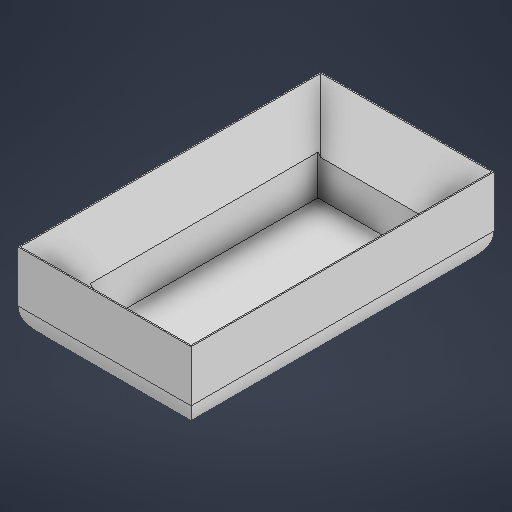
# Autodesk Inventor part: мыльница
Saved by Autodesk Inventor 2025 (Build 290162000, 162)
## iProperties
Created: 2024-12-03
Part Number: мыльница
Material: Типовые
Document SubType Name: Modeling
Designer: GameHD
Density: 1 g/cm^3
Appearance: По умолчанию
Author: GameHD
Autodesk Inventor part; units mm, degrees
ref_plane "YZ Plane" through (0, 0, 0) normal (1, 0, 0) x (0, 1, 0)
ref_plane "XZ Plane" through (0, 0, 0) normal (0, 1, 0) x (-1, 0, 0)
ref_plane "XY Plane" through (0, 0, 0) normal (0, 0, 1) x (1, 0, 0)
sketch "Эскиз1" plane through (0, 0, 0) normal (0, 0, 1) x (1, 0, 0)
  line L0 (-19.75, -19.75) -> (19.75, -19.75)
  line L1 (19.75, -19.75) -> (19.75, 19.75)
  line L2 (19.75, 19.75) -> (-19.75, 19.75)
  line L3 (-19.75, 19.75) -> (-19.75, -19.75)
  line L4 (-19.75, -19.75) -> (19.75, 19.75) construction
  line L5 (19.75, -19.75) -> (-19.75, 19.75) construction
  line L6 (-35, -35) -> (35, -35)
  line L7 (35, -35) -> (35, 35)
  line L8 (35, 35) -> (-35, 35)
  line L9 (-35, 35) -> (-35, -35)
  line L10 (-35, -35) -> (35, 35) construction
  line L11 (35, -35) -> (-35, 35) construction
  line L12 (-19.75, 19.75) -> (-35, 19.75)
  line L13 (19.75, 19.75) -> (35, 19.75)
  point P0 (0, 0)
  dimension "d0" = 39.5
  dimension "d1" = 39.5
  dimension "d2" = 70
  dimension "d3" = 70
  constraints: 28 end point, 4 midpoint, 4 parallel, 3 perpendicular, 3 point on line, 2 horizontal
  measures "d0" distance of L2.end L1.end
  measures "d1" distance of L1.end L0.end
  measures "d2" distance of L8.end L7.end
  measures "d3" distance of L8.end L6.start
extrude "Выдавливание1" add sketch "Эскиз1" along normal blind 92 contours L0 L1 L13 L7 L6 L9 L12 L3
sketch "Эскиз2" plane through (0, 0, 0) normal (0, 0, -1) x (-1, 0, 0)
  line L0 (-19.75, -19.75) -> (19.75, -19.75) projected
  line L1 (-19.75, 19.75) -> (-19.75, -19.75) projected
  line L2 (-35, 19.75) -> (-19.75, 19.75) projected
  line L3 (-35, -35) -> (-35, 19.75) projected
  line L4 (35, -35) -> (-35, -35) projected
  line L5 (35, 19.75) -> (35, -35) projected
  line L6 (19.75, 19.75) -> (35, 19.75) projected
  line L7 (19.75, -19.75) -> (19.75, 19.75) projected
  line L8 (-19.75, 19.75) -> (19.75, 19.75)
  point P0 (0, 0)
  constraints: 2 end point, 1 horizontal
extrude "Выдавливание2" add sketch "Эскиз2" along normal blind 15.25
sketch "Эскиз3" plane through (0, 0, 92) normal (0, 0, 1) x (1, 0, 0)
  line L0 (19.75, -19.75) -> (-19.75, -19.75) projected
  line L1 (-19.75, -19.75) -> (-19.75, 19.75) projected
  line L2 (-19.75, 19.75) -> (-35, 19.75) projected
  line L3 (-35, 19.75) -> (-35, -35) projected
  line L4 (-35, -35) -> (35, -35) projected
  line L5 (35, -35) -> (35, 19.75) projected
  line L6 (35, 19.75) -> (19.75, 19.75) projected
  line L7 (19.75, 19.75) -> (19.75, -19.75) projected
  line L8 (-19.75, 19.75) -> (19.75, 19.75) projected
  point P0 (0, 0)
extrude "Выдавливание3" add sketch "Эскиз3" along normal blind 15.25
sketch "Эскиз4" plane through (-35, -35, -15.25) normal (-1, 0, 0) x (0, 0, 1)
  line L0 (0, 54.75) -> (200, 54.75)
  line L1 (200, 54.75) -> (200, 44.75)
  line L2 (200, 44.75) -> (0, 44.75)
  line L3 (0, 44.75) -> (0, 54.75)
  dimension "d12" = 200
  dimension "d13" = 10
  constraints: 8 end point, 2 parallel, 1 horizontal, 1 perpendicular
  measures "d12" distance of L1.end L2.end
  measures "d13" distance of L0.end L1.end
extrude "Выдавливание4" cut sketch "Эскиз4" against normal through all
chamfer "Фаска1" distance 14.7625 angle 45 4 edges at (0, 9.75, 92) (19.75, 9.75, 46) (-19.75, 9.75, 46) (0, 9.75, 0)
sketch "Эскиз5" plane through (-35, -35, -15.25) normal (0, -1, 0) x (1, 0, 0)
  line L0 (70, 0) -> (70, 122.5) projected
  line L1 (0, 122.5) -> (70, 122.5) projected
  line L2 (0, 0) -> (0, 122.5) projected
  line L3 (70, 0) -> (0, 0) projected
  point P0 (35, 15.25)
extrude "Выдавливание5" cut sketch "Эскиз5" against normal blind 12.05
fillet "Сопряжение1" radius 12 4 edges at (35, -22.95, 46) (0, -22.95, 107.25) (0, -22.95, -15.25) (-35, -22.95, 46)
sketch "Эскиз6" plane through (-19.75, -19.75, 0) normal (0, 1, 0) x (1, 0, 0)
  line L0 (39.5, 0) -> (0, 0) projected
  line L1 (0, 0) -> (0, -92) projected
  line L2 (39.5, -92) -> (0, -92) projected
  line L3 (39.5, 0) -> (39.5, -92) projected
  line L4 (-1.25, -92) -> (-1.25, 0)
  line L5 (-1.25, 0) -> (40.75, 0)
  line L6 (40.75, 0) -> (40.75, -92)
  line L7 (40.75, -92) -> (-1.25, -92)
  line L8 (-1.25, -92) -> (40.75, 0) construction
  line L9 (-1.25, 0) -> (40.75, -92) construction
  point P0 (19.75, 0)
  point P1 (19.75, -46)
  dimension "d22" = 42
  constraints: 12 end point, 2 midpoint, 2 parallel, 2 perpendicular
  measures "d22" distance of L4.end L5.end
extrude "Выдавливание6" cut sketch "Эскиз6" along normal through all
